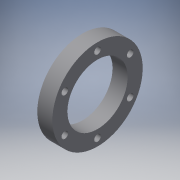
# Autodesk Inventor part: Motor Spacer
Saved by Autodesk Inventor 2019.4 (Build 234330000, 330)
## iProperties
Created: 2020-01-06
Part Number: Motor Spacer
Material: Aluminum 6061
Document SubType Name: Modeling
Designer: Mark
Mass: 29.9612 g
Surface Area: 59.3736 cm^2
Volume: 11.0967 cm^3
Density: 2.7 g/cm^3
Appearance: Aluminum - Flat
Author: Mark
Autodesk Inventor part; units mm, degrees
ref_plane "YZ Plane" through (0, 0, 0) normal (1, 0, 0) x (0, 1, 0)
ref_plane "XZ Plane" through (0, 0, 0) normal (0, 1, 0) x (-1, 0, 0)
ref_plane "XY Plane" through (0, 0, 0) normal (0, 0, 1) x (1, 0, 0)
sketch "Sketch1" plane through (0, 0, 0) normal (1, 0, 0) x (0, 1, 0)
  circle A0 centre (0, 0) radius 20
  circle A1 centre (0, 0) radius 25.4 construction
  circle A2 centre (25.4, 0) radius 2.2
  circle A3 centre (0, 0) radius 25.4 construction
  circle A4 centre (12.7, 21.997) radius 2.2
  circle A5 centre (0, 0) radius 25.4 construction
  circle A6 centre (-12.7, 21.997) radius 2.2
  circle A7 centre (0, 0) radius 25.4 construction
  circle A8 centre (-25.4, 0) radius 2.2
  circle A9 centre (0, 0) radius 25.4 construction
  circle A10 centre (-12.7, -21.997) radius 2.2
  circle A11 centre (0, 0) radius 25.4 construction
  circle A12 centre (12.7, -21.997) radius 2.2
  circle A13 centre (0, 0) radius 30
  dimension "d1" = 50.8
  dimension "d0" = 40
  dimension "d2" = 4.4
  dimension "d5" = 360
  dimension "d7" = 60
  constraints: 8 centre point, 3 coincident, 2 horizontal alignment, 41 other
  measures "d0" diameter of A0
  measures "d2" diameter of A2
  measures "d7" diameter of A13
extrude "Extrusion1" add sketch "Sketch1" along normal blind 7.5
body "Solid1"
